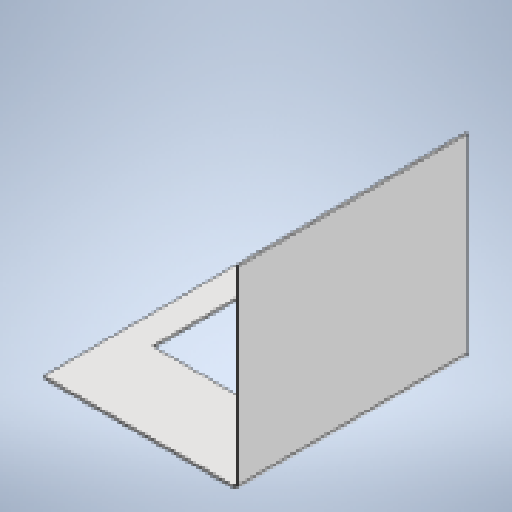
# Autodesk Inventor part: MNT-CDF-503  main tube 1
Saved by Autodesk Inventor 2025.1 (Build 291241020, 241B)
## iProperties
Created: 2025-01-13
Part Number: MNT-CDF-503  main tube 1
Material: Stainless Steel
Description: DIE16(5)|\ 90°|corrY -___°|X_____|bom___
Document SubType Name: Sheet Metal
Designer: user
Stock Number: МОО 305 шпангоут борт
Mass: 1762.25 g
Surface Area: 2283.33 cm^2
Volume: 220.281 cm^3
Density: 8 g/cm^3
Sheet Metal Rule: AISI304 2mm Die16
Sheet Metal Width: 0.000 mm
Sheet Metal Length: 0.000 mm
Sheet Metal Area: 0.000 mm^2
Appearance: Default
БОРТ_стрингер_3_высота: 63.000 mm
БОРТ_стрингер_4_высота: 48.000 mm
БОРТ_стрингер_5_высота: 54.000 mm
БОРТ_стрингер_6_высота: 81.000 mm
РЕБРА_глубина_паза: 28.000 mm
РЕБРА_вырез_на_полке: 5,000 mm
РЕБРА_полка: 20,000 mm
Author: user
Autodesk Inventor part; units mm, degrees
ref_plane "YZ Plane" through (0, 0, 0) normal (1, 0, 0) x (0, 1, 0)
ref_plane "XZ Plane" through (0, 0, 0) normal (0, 1, 0) x (-1, 0, 0)
ref_plane "XY Plane" through (0, 0, 0) normal (0, 0, 1) x (1, 0, 0)
sketch "Sketch1" plane through (0, 0, 0) normal (0, 0, 1) x (1, 0, 0)
  line L0 (-77.5, -60) -> (77.5, -60)
  line L1 (77.5, -60) -> (77.5, 60)
  line L2 (77.5, 60) -> (-77.5, 60)
  line L3 (-77.5, 60) -> (-77.5, -60)
  line L4 (-77.5, -60) -> (77.5, 60) construction
  line L5 (77.5, -60) -> (-77.5, 60) construction
  point P0 (0, 0)
  dimension "d154" = 155
  dimension "d155" = 120
  measures "d154" distance of L1.end L2.end
  measures "d155" distance of L0.end L1.end
extrude "Plate3" add sketch "Sketch1" along normal blind 2
sketch "Sketch7" plane through (75.5, 60, 0) normal (1, 0, 0) x (0, 1, 0)
  line L0 (-120, 0) -> (0, 0)
  line L1 (0, 0) -> (0, 155)
  line L2 (0, 155) -> (-120, 155)
  line L3 (-120, 155) -> (-120, 0)
  constraints: 6 end point, 1 horizontal, 1 perpendicular, 1 vertical
edge flange "Flange3" height 155 angle 90 thickness 2 bend radius 2.75 thickness toward (1, 0, 0) relief round relief width 2 relief depth 1 edges at (77.5, 0, 2) wall of the first edge with corners at (75.5, -60, 0) (75.5, 60, 0) (75.5, 60, 155) (75.5, -60, 155)
bend "Bend3"
corner "Corner3"
sketch "Sketch8" plane through (0, 0, 2) normal (0, 0, 1) x (1, 0, 0)
  line L0 (60, 50) -> (-60, 50)
  line L1 (-60, 50) -> (-60, -30)
  line L2 (-60, -30) -> (60, -30)
  line L3 (60, -30) -> (60, 50)
  line L4 (60, 50) -> (-60, -30) construction
  line L5 (-60, 50) -> (60, -30) construction
  line L6 (-77.5, 60) -> (72.75, 60) projected
  point P0 (0, 0)
  point P1 (0, 10)
  dimension "d166" = 120
  dimension "d167" = 80
  dimension "d168" = 10
  constraints: 12 end point, 2 midpoint, 2 parallel, 1 horizontal, 1 perpendicular, 1 vertical alignment
  measures "d166" distance of L2.end L1.end
  measures "d167" distance of L1.end L0.end
  measures "d168" distance between parallel lines of L0 L6
extrude "Cut1" cut sketch "Sketch8" against normal blind 2
equation "\"БОРТ_стрингер_3_высота\" = 63"
equation "\"БОРТ_стрингер_4_высота\" = 48"
equation "\"БОРТ_стрингер_5_высота\" = 54"
equation "\"БОРТ_стрингер_6_высота\" = 81"
body "Solid2"
